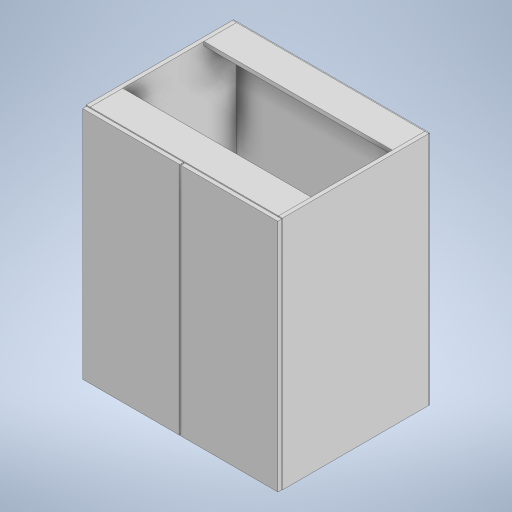
# Autodesk Inventor part: Base Cabinet 3
Saved by Autodesk Inventor 2024 (Build 280153000, 153)
## iProperties
Created: 2023-06-24
Part Number: Base Cabinet 3
Material: Generic
Document SubType Name: Modeling
Designer: 69
Density: 1 g/cm^3
Appearance: Default
Author: 69
Autodesk Inventor part; units mm, degrees
ref_plane "YZ Plane" through (0, 0, 0) normal (1, 0, 0) x (0, 1, 0)
sketch "Sketch1" plane through (0, 0, 0) normal (0, 0, 1) x (1, 0, 0)
  line L0 (-1498, 0) -> (1498, 0) construction
  line L1 (-1498, 0) -> (-898, 0)
  line L2 (-898, 0) -> (-898, 2068)
  line L3 (-898, 2068) -> (-1498, 2068)
  line L4 (-1498, 2068) -> (-1498, 0)
  line L5 (-898, 0) -> (-498, 0)
  line L6 (-498, 0) -> (-498, 816)
  line L7 (-498, 816) -> (-898, 816)
  line L8 (-898, 816) -> (-898, 0)
  line L9 (-498, 0) -> (102, 0)
  line L10 (102, 0) -> (102, 816)
  line L11 (102, 816) -> (-498, 816)
  line L12 (-498, 816) -> (-498, 0)
  line L13 (102, 0) -> (698, 0)
  line L14 (698, 0) -> (698, 668)
  line L15 (698, 668) -> (102, 668)
  line L16 (102, 668) -> (102, 0)
  line L17 (698, 0) -> (1498, 0)
  line L18 (1498, 0) -> (1498, 816)
  line L19 (1498, 816) -> (698, 816)
  line L20 (698, 816) -> (698, 0)
  line L21 (-1498, 0) -> (1498, 0)
  line L22 (1498, 0) -> (1498, 96)
  line L23 (1498, 96) -> (-1498, 96)
  line L24 (-1498, 96) -> (-1498, 0)
  line L25 (-898, 816) -> (1498, 816)
  line L26 (1498, 816) -> (1498, 832)
  line L27 (1498, 832) -> (-898, 832)
  line L28 (-898, 832) -> (-898, 816)
  line L29 (-898, 1972) -> (-498, 1972)
  line L30 (-498, 1972) -> (-498, 1372)
  line L31 (-498, 1372) -> (-898, 1372)
  line L32 (-898, 1372) -> (-898, 1972)
  line L33 (698, 1972) -> (1498, 1972)
  line L34 (1498, 1972) -> (1498, 1372)
  line L35 (1498, 1372) -> (698, 1372)
  line L36 (698, 1372) -> (698, 1972)
  line L37 (698, 1372) -> (98, 1372)
  line L38 (98, 1372) -> (98, 1972)
  line L39 (98, 1972) -> (698, 1972)
  line L40 (698, 1972) -> (698, 1372)
  line L41 (-498, 1372) -> (98, 1372)
  line L42 (-498, 1372) -> (-275, 1637.7611)
  line L43 (98, 1372) -> (-125, 1637.7611)
  line L44 (-275, 1637.7611) -> (-125, 1637.7611)
  line L45 (-125, 1637.7611) -> (-125, 2068)
  line L46 (-125, 2068) -> (-275, 2068)
  line L47 (-275, 2068) -> (-275, 1637.7611)
  line L48 (1098, 816) -> (1098, 96)
  line L49 (-198, 816) -> (-198, 96)
  line L50 (-898, 668) -> (-498, 668)
  line L51 (-1498, 520) -> (-898, 520)
  line L52 (-1498, 1579) -> (-898, 1579)
  line L53 (398, 1972) -> (398, 1372)
  line L54 (1098, 1972) -> (1098, 1372)
  line L55 (698, 1876) -> (1498, 1876)
  line L56 (698, 1468) -> (1498, 1468)
  line L57 (-1498, 1049.5) -> (-898, 1049.5)
  point P0 (0, 0)
  point P1 (0, 0)
  point P2 (0, 0)
  point P3 (-198, 816)
  point P4 (0, 0)
  dimension "d0" = 2996
  dimension "d1" = 600
  dimension "d2" = 2068
  dimension "d3" = 400
  dimension "d4" = 816
  dimension "d5" = 600
  dimension "d6" = 816
  dimension "d7" = 596
  dimension "d8" = 668
  dimension "d9" = 800
  dimension "d10" = 816
  dimension "d11" = 96
  dimension "d12" = 16
  dimension "d13" = 400
  dimension "d14" = 600
  dimension "d15" = 96
  dimension "d16" = 800
  dimension "d17" = 600
  dimension "d18" = 600
  dimension "d19" = 600
  dimension "d20" = 50
  dimension "d21" = 150
  dimension "d22" = 148
  dimension "d23" = 1059
  dimension "d24" = 96
  dimension "d25" = 96
  dimension "d26" = 529.5
  constraints: 116 end point, 22 parallel, 18 point on line, 17 perpendicular, 14 horizontal, 8 midpoint, 4 coincident, 4 horizontal alignment, 2 vertical alignment, 1 equal length
  measures "d0" distance of L0.start L0.end
  measures "d1" distance of L3.end L2.end
  measures "d2" distance of L2.end L1.end
  measures "d3" distance of L7.end L6.end
  measures "d4" distance of L6.end L5.end
  measures "d5" distance of L11.end L10.end
  measures "d6" distance of L9.end L10.end
  measures "d7" distance of L15.end L14.end
  measures "d8" distance of L14.end L13.end
  measures "d9" distance of L19.end L18.end
  measures "d10" distance of L18.end L17.end
  measures "d11" distance of L22.end L21.end
  measures "d12" distance of L26.end L25.end
  measures "d13" distance of L30.end L31.end
  measures "d14" distance of L29.end L30.end
  measures "d15" distance between parallel lines of L3 L29
  measures "d16" distance of L34.end L35.end
  measures "d17" distance of L33.end L34.end
  measures "d18" distance of L38.end L39.end
  measures "d19" distance of L37.end L38.end
  measures "d20" angle of L41 L42
  measures "d21" distance of L43.end L42.end
  measures "d22" distance of L50.start L51.end
  measures "d23" distance between parallel lines of L51 L52
  measures "d24" distance of L33.start L55.start
  measures "d25" distance of L56.start L35.end
  measures "d26" distance between parallel lines of L51 L57
ref_plane "Work Plane1" through (1498, 96, 0) normal (0, 1, 0) x (-1, 0, 0)
sketch "Sketch2" plane through (1498, 96, 0) normal (0, 1, 0) x (-1, 0, 0)
  line L0 (1996, 0) -> (1396, 0)
  line L1 (1396, 0) -> (1396, 460)
  line L2 (1396, 460) -> (1996, 460)
  line L3 (1996, 460) -> (1996, 0)
  line L4 (1984, 448) -> (1408, 448)
  line L5 (1408, 448) -> (1408, 12)
  line L6 (1408, 12) -> (1984, 12)
  line L7 (1984, 12) -> (1984, 448)
  line L8 (1984, 12) -> (1984, 0)
  line L9 (1408, 12) -> (1408, 0)
  line L10 (1408, 448) -> (1396, 448)
  line L11 (1984, 448) -> (1996, 448)
  point P0 (1498, 0)
  point P1 (1996, 0)
  point P2 (1396, 0)
  dimension "d28" = 460
  dimension "d29" = 12
  constraints: 24 end point, 5 perpendicular, 5 point on line, 4 parallel, 1 coincident, 1 horizontal, 3 other
  measures "d28" distance of L0.end L1.end
  measures "d29" distance between parallel lines of L2 L4
extrude "Extrusion1" add sketch "Sketch2" along normal up to surface (720 mm away) contours L0 L8 L7 L11 L3 | L0 L1 L10 L5 L9
extrude "Extrusion2" add sketch "Sketch2" along normal up to surface (720 mm away) separate body contours L11 L4 L10 L1 L2 L3
split body "Split1" sketch "Sketch1" result two bodies bodies 2 curves L49 first body at (2, 336, 459.5)
sketch "Sketch3" plane through (1498, 96, 0) normal (0, 1, 0) x (-1, 0, 0)
  line L0 (1996, 0) -> (1996, 448) projected
  line L1 (1996, 0) -> (1396, 0)
  line L2 (1396, 0) -> (1396, -3)
  line L3 (1396, -3) -> (1996, -3)
  line L4 (1996, -3) -> (1996, 0)
  point P0 (1498, 0)
  dimension "d34" = 3
  constraints: 8 end point, 2 parallel, 1 coincident, 1 horizontal, 1 perpendicular
  measures "d34" distance of L1.end L2.end
extrude "Extrusion3" add sketch "Sketch3" along normal up to surface (720 mm away) separate body
sketch "Sketch4" plane through (1498, 96, 0) normal (0, 1, 0) x (-1, 0, 0)
  line L0 (1984, 0) -> (1984, 448) projected
  line L1 (1396, 0) -> (1996, 0) projected
  line L2 (1408, 448) -> (1408, 0) projected
  line L3 (1996, 448) -> (1696, 448) projected
  line L4 (1696, 448) -> (1396, 448) projected
  point P0 (1498, 0)
extrude "Extrusion4" add sketch "Sketch4" along normal blind 12 separate body
ref_plane "Work Plane2" through (102, 816, 336) normal (0, -1, 0) x (0, 0, 1)
sketch "Sketch5" plane through (102, 816, 336) normal (0, -1, 0) x (0, 0, 1)
  line L0 (-336, 588) -> (112, 588) projected
  line L1 (112, 12) -> (-336, 12) projected
  line L2 (-336, 0) -> (-336, 600) projected
  line L3 (112, 600) -> (112, 300) projected
  line L4 (112, 300) -> (112, 0) projected
  line L5 (-236, 588) -> (-236, 12)
  line L6 (12, 588) -> (12, 12)
  point P0 (-336, 102)
  dimension "d39" = 100
  dimension "d40" = 100
  constraints: 4 end point, 4 point on line, 2 perpendicular
  measures "d39" distance between parallel lines of L5 L2
  measures "d40" distance between parallel lines of L4 L6
extrude "Extrusion5" add sketch "Sketch5" along normal blind 12 separate body contours L0 L5 L1 L2 | L0 L3 L4 L1 L6
sketch "Sketch6" plane through (102, 96, 460) normal (0, 0, 1) x (1, 0, 0)
  line L0 (-600, 720) -> (-300, 720) projected
  line L1 (0, 0) -> (-300, 0) projected
  line L2 (-301.5, 720) -> (-298.5, 720)
  line L3 (-298.5, 720) -> (-298.5, 0)
  line L4 (-298.5, 0) -> (-301.5, 0)
  line L5 (-301.5, 0) -> (-301.5, 720)
  line L6 (-300, 0) -> (-300, 720) projected
  point P0 (-102, -96)
  point P1 (-300, 720)
  dimension "d43" = 1.5
  dimension "d44" = 1.5
  constraints: 8 end point, 2 parallel, 2 point on line, 1 horizontal, 1 perpendicular
  measures "d43" distance between parallel lines of L6 L3
  measures "d44" distance between parallel lines of L6 L5
extrude "Extrusion6" cut sketch "Sketch6" against normal blind 12 bodies 3 4
sketch "Sketch7" plane through (-498, 96, 0) normal (0, 0, 1) x (1, 0, 0)
  line L0 (12, 0) -> (12, 720) projected
  line L1 (588, 0) -> (588, 720) projected
  line L2 (12, 366) -> (588, 366)
  line L3 (588, 366) -> (588, 354)
  line L4 (588, 354) -> (12, 354)
  line L5 (12, 354) -> (12, 366)
  line L6 (12, 12) -> (588, 12) projected
  point P0 (498, -96)
  point P1 (12, 354)
  dimension "d47" = 342
  dimension "d48" = 12
  constraints: 8 end point, 2 parallel, 2 point on line, 1 horizontal, 1 perpendicular
  measures "d47" distance between parallel lines of L6 L4
  measures "d48" distance between parallel lines of L4 L2
extrude "Extrusion7" add sketch "Sketch7" along normal up to surface (448 mm away) separate body contours L0 L2 L1 L4
sketch "Sketch9" plane through (-498, 96, 460) normal (0, 0, 1) x (1, 0, 0)
  line L0 (0, 0) -> (0, 720) projected
  line L1 (600, 0) -> (600, 720) projected
  line L2 (0, 720) -> (600, 720)
  line L3 (600, 720) -> (600, 717)
  line L4 (600, 717) -> (0, 717)
  line L5 (0, 717) -> (0, 720)
  line L6 (0, 0) -> (298.5, 0) projected
  line L7 (0, 717) -> (1.5, 717)
  line L8 (1.5, 717) -> (1.5, 0)
  line L9 (1.5, 0) -> (0, 0)
  line L10 (0, 0) -> (0, 717)
  line L11 (600, 717) -> (598.5, 717)
  line L12 (598.5, 717) -> (598.5, 0)
  line L13 (598.5, 0) -> (600, 0)
  line L14 (600, 0) -> (600, 717)
  point P0 (498, -96)
  dimension "d55" = 3
  dimension "d56" = 1.5
  dimension "d57" = 1.5
  constraints: 24 end point, 6 parallel, 3 horizontal, 3 perpendicular, 3 point on line
  measures "d55" distance of L1.end L3.end
  measures "d56" distance between parallel lines of L1 L12
  measures "d57" distance between parallel lines of L0 L8
extrude "Extrusion9" cut sketch "Sketch9" against normal blind 12 bodies 4 3
